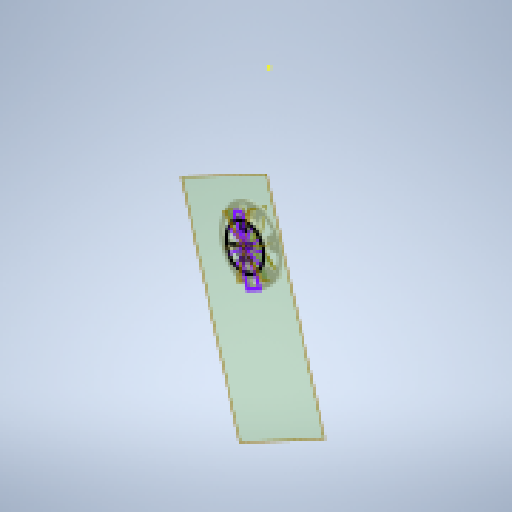
# Autodesk Inventor part: Part48
Saved by Autodesk Inventor 2023.1 (Build 271208000, 208)
## iProperties
Created: 2022-12-24
Part Number: Part48
Material: Generic
Document SubType Name: Modeling
Designer: USER
Density: 1 g/cm^3
Appearance: Default
Author: USER
## iProperties of the stored document Part48_3DPrint.ipt
Created: 2022-12-24
Part Number: Part48_3DPrint
Material: Generic
Document SubType Name: Modeling
Designer: USER
Density: 1 g/cm^3
Appearance: Default
Author: USER
Autodesk Inventor part; units mm, degrees
ref_plane "YZ Plane" through (0, 0, 0) normal (1, 0, 0) x (0, 1, 0)
ref_plane "XZ Plane" through (0, 0, 0) normal (0, 1, 0) x (-1, 0, 0)
ref_plane "XY Plane" through (0, 0, 0) normal (0, 0, 1) x (1, 0, 0)
ref_plane "Work Plane1" through (4.516, -244.3123, 193.8348) normal (0.0815899, -0.1423035, -0.9864547) x (-0.8818057, -0.4715874, -0.0049043)
sketch "Sketch1" plane through (4.516, -244.3123, 193.8348) normal (0.0815899, -0.1423035, -0.9864547) x (-0.8818057, -0.4715874, -0.0049043)
  circle A0 centre (-7.3856, 63.5963) radius 27.5
  circle A1 centre (-7.3856, 63.5963) radius 29.5
  line L0 (-7.3856, 63.5963) -> (21.2381, 70.733)
  line L1 (-7.3856, 63.5963) -> (22.1144, 63.5963) construction
  line L2 (-7.3856, 63.5963) -> (21.2381, 56.4596)
  line L3 (-7.3856, 63.5963) -> (-36.0093, 56.4596)
  line L4 (-7.3856, 63.5963) -> (11.5206, 86.2415)
  line L5 (-7.3856, 63.5963) -> (13.8349, 43.1038)
  line L6 (-7.3856, 63.5963) -> (-27.8852, 42.3827)
  line L7 (-7.3856, 63.5963) -> (-27.3405, 85.323)
  line L8 (-7.3856, 63.5963) -> (-36.0093, 70.733)
  line L9 (1.9118, 35.5997) -> (-7.3856, 63.5963)
  line L10 (-7.3856, 63.5963) -> (-14.5223, 34.9725)
  line L11 (-7.3856, 63.5963) -> (-3.5711, 92.8486)
  line L12 (-7.3856, 63.5963) -> (-13.8284, 92.3841)
  line L13 (1.2815, 37.4978) -> (-3.8297, 90.8654)
  line L14 (-14.0384, 36.9131) -> (-13.3916, 90.4324)
  line L15 (1.2815, 37.4978) -> (1.2815, 20.7047)
  line L16 (1.2815, 20.7047) -> (-15.5202, 20.7047)
  line L17 (-15.5202, 20.7047) -> (-14.0384, 36.9131)
  line L18 (-16.0526, 37.4978) -> (-17.5191, 18.7055)
  line L19 (-17.5191, 18.7055) -> (4.7638, 18.7055)
  line L20 (4.7638, 18.7055) -> (3.3138, 38.263)
  line L21 (-3.5711, 92.8486) -> (-4.046, 99.2535)
  line L22 (-4.046, 99.2535) -> (-6.8936, 100.1817)
  line L23 (-6.8936, 100.1817) -> (-9.9321, 100.1817)
  line L24 (-9.9321, 100.1817) -> (-13.8284, 98.8878)
  line L25 (-13.8284, 98.8878) -> (-13.8284, 92.3841)
  line L26 (-15.3417, 92.0031) -> (-15.3417, 99.2535)
  line L27 (-15.3417, 99.2535) -> (-9.9193, 101.5782)
  line L28 (-9.9193, 101.5782) -> (-7.0854, 101.5782)
  line L29 (-7.0854, 101.5782) -> (-3.122, 101.2612)
  line L30 (-3.122, 101.2612) -> (-0.9428, 92.3841)
  point P0 (-110.2818, 246.4946)
  point P1 (-14.0384, 36.9131)
  point P2 (-13.3916, 90.4324)
  point P3 (-3.8297, 90.8654)
  point P4 (1.2815, 37.4978)
  point P5 (-25.9876, 83.85)
  point P6 (-34.0687, 70.2491)
  point P7 (-34.0687, 56.9434)
  point P8 (-26.4954, 43.8209)
  point P9 (12.3963, 44.4932)
  point P10 (19.2975, 56.9434)
  point P11 (19.2975, 70.2491)
  point P12 (10.2388, 84.7062)
  point P13 (-14.2225, 34.8995)
  point P14 (-16.2126, 35.4478)
  point P15 (3.4693, 36.1659)
  point P16 (1.2815, 35.3982)
  dimension "d1" = 59
  dimension "d0" = 55
  dimension "d2" = 14
  constraints: 62 end point, 6 point on circle, 5 point on line, 4 parallel, 3 horizontal, 2 vertical, 1 centre point, 1 coincident, 1 equal length, 17 other
  measures "d0" diameter of A0
  measures "d2" angle of L1 L0
extrude "Extrusion1" add sketch "Sketch1" along normal blind 4 contours L11 A1 L4 A0 | A0 L7 A1 L12 | L4 A1 L0 A0 | A0 L8 A1 L7 | L0 A1 L2 A0 | A0 L20 A1 L9 | L10 A1 L18 A0 | A0 L3 A1 L8 | L2 A1 L5 A0 | A0 L6 A1 L3 | L5 A1 L20 A0 | A0 L18 A1 L6
extrude "Extrusion2" add sketch "Sketch1" along normal blind 8 contours L11 A1 L4 A0 | A0 L7 A1 L12 | L0 A1 L2 A0 | A0 L20 A1 L9 | L10 A1 L18 A0 | A0 L3 A1 L8 | L5 A1 L20 A0 | A0 L18 A1 L6
ref_plane "Work Plane2" through (-18.1856, -186.0532, 179.4979) normal (0.9966606, 0.0148992, 0.0802847) x (-0.0815899, 0.1423035, 0.9864547)
sketch "Sketch3" plane through (5.1687, -245.4507, 185.9432) normal (0.0815899, -0.1423035, -0.9864547) x (0.8818057, 0.4715874, 0.0049043)
  arc A0 (36.0093, -70.733) -> (36.0093, -56.4596) centre (7.3856, -63.5963) ccw projected
  line L0 (36.0093, -56.4596) -> (34.0687, -56.9434) projected
  arc A1 (34.0687, -70.2491) -> (34.0687, -56.9434) centre (7.3856, -63.5963) ccw projected
  line L1 (34.0687, -70.2491) -> (36.0093, -70.733) projected
  arc A2 (26.4954, -43.8209) -> (14.0384, -36.9131) centre (7.3856, -63.5963) ccw projected
  line L2 (26.4954, -43.8209) -> (27.8852, -42.3827) projected
  arc A3 (27.8852, -42.3827) -> (14.5223, -34.9725) centre (7.3856, -63.5963) ccw projected
  line L3 (14.5223, -34.9725) -> (14.0384, -36.9131) projected
  arc A4 (13.8284, -92.3841) -> (27.3405, -85.323) centre (7.3856, -63.5963) ccw projected
  line L4 (27.3405, -85.323) -> (25.9876, -83.85) projected
  arc A5 (13.3916, -90.4324) -> (25.9876, -83.85) centre (7.3856, -63.5963) ccw projected
  line L5 (13.3916, -90.4324) -> (13.8284, -92.3841) projected
  arc A6 (-10.2388, -84.7062) -> (3.8297, -90.8654) centre (7.3856, -63.5963) ccw projected
  line L6 (-10.2388, -84.7062) -> (-11.5206, -86.2415) projected
  arc A7 (-11.5206, -86.2415) -> (3.5711, -92.8486) centre (7.3856, -63.5963) ccw projected
  line L7 (3.5711, -92.8486) -> (3.8297, -90.8654) projected
  arc A8 (-21.2381, -56.4596) -> (-21.2381, -70.733) centre (7.3856, -63.5963) ccw projected
  line L8 (-21.2381, -70.733) -> (-19.2975, -70.2491) projected
  arc A9 (-19.2975, -56.9434) -> (-19.2975, -70.2491) centre (7.3856, -63.5963) ccw projected
  line L9 (-19.2975, -56.9434) -> (-21.2381, -56.4596) projected
  arc A10 (-1.9118, -35.5997) -> (-13.8349, -43.1038) centre (7.3856, -63.5963) ccw projected
  line L10 (-13.8349, -43.1038) -> (-12.3963, -44.4932) projected
  arc A11 (-1.2815, -37.4978) -> (-12.3963, -44.4932) centre (7.3856, -63.5963) ccw projected
  line L11 (-1.2815, -37.4978) -> (-1.9118, -35.5997) projected
  circle A12 centre (7.3856, -63.5963) radius 42.2209
  line L12 (-13.8349, -43.1038) -> (-22.6179, -33.8911)
  arc A13 (-1.9118, -35.5997) -> (3.5711, -92.8486) centre (7.3856, -63.5963) ccw projected
  line L13 (-1.9118, -35.5997) -> (-1.9118, -22.4118)
  arc A14 (27.8852, -42.3827) -> (14.5223, -34.9725) centre (7.3856, -63.5963) ccw projected
  line L14 (14.5223, -34.9725) -> (14.5223, -21.9829)
  line L15 (27.8852, -42.3827) -> (37.2658, -33.7671)
  line L16 (36.0093, -56.4596) -> (48.3523, -53.3821)
  line L17 (36.0093, -70.733) -> (48.3523, -73.8104)
  line L18 (27.3405, -85.323) -> (35.9454, -94.692)
  line L19 (13.8284, -92.3841) -> (14.5223, -105.2096)
  line L20 (3.5711, -92.8486) -> (3.5711, -105.6445)
  line L21 (-11.5206, -86.2415) -> (-20.7695, -95.0589)
  line L22 (-21.2381, -70.733) -> (-33.9344, -72.2715)
  line L23 (-21.2381, -56.4596) -> (-33.5811, -53.3821)
  circle A15 centre (7.3856, -63.5963) radius 46.8447
  circle A16 centre (-7.8498, -97.5441) radius 2.1
  circle A17 centre (-30.2116, -64.0433) radius 2.1
  circle A18 centre (-13.2655, -31.9742) radius 2.1
  circle A19 centre (25.3852, -30.0564) radius 2.1
  circle A20 centre (45.1864, -63.6105) radius 2.1
  circle A21 centre (25.0924, -96.3018) radius 2.1
  circle A22 centre (25.0924, -96.3018) radius 1.65
  circle A23 centre (45.1864, -63.6105) radius 1.65
  circle A24 centre (25.3852, -30.0564) radius 1.65
  circle A25 centre (-13.2655, -31.9742) radius 1.65
  circle A26 centre (-30.2116, -64.0433) radius 1.65
  circle A27 centre (-7.8498, -97.5441) radius 1.65
  point P0 (110.2818, -246.4946)
  dimension "d31" = 3.3
  dimension "d32" = 3.3
  dimension "d33" = 3.3
  dimension "d34" = 3.3
  dimension "d35" = 3.3
  dimension "d36" = 3.3
  constraints: 24 end point, 13 centre point, 8 coincident, 2 parallel, 2 perpendicular, 2 point on line, 1 point on circle, 1 vertical, 26 other
  measures "d31" diameter of A22
  measures "d32" diameter of A23
  measures "d33" diameter of A24
  measures "d34" diameter of A25
  measures "d35" diameter of A26
  measures "d36" diameter of A27
ref_plane "Work Plane3" through (-18.1856, -186.0532, 179.4979) normal (-0.4645017, 0.8702615, -0.1639608) x (0.0815899, -0.1423035, -0.9864547)
ref_plane "Work Plane4" through (-18.5119, -185.484, 183.4438) normal (-0.5459087, -0.8344608, 0.075225) x (-0.0815899, 0.1423035, 0.9864547)
ref_plane "Work Plane5" through (-18.5119, -185.484, 183.4438) normal (0.9937194, -0.064436, 0.0914861) x (0.0815899, -0.1423035, -0.9864547)
ref_plane "Work Plane6" through (-18.1856, -186.0532, 179.4979) normal (0.4645017, -0.8702615, 0.1639608) x (0.0815899, -0.1423035, -0.9864547)
ref_plane "Work Plane7" through (-18.1856, -186.0532, 179.4979) normal (-0.6214967, -0.7810177, 0.0612635) x (0.0815899, -0.1423035, -0.9864547)
extrude "Extrusion7" add sketch "Sketch3" along normal blind 2.0625 contours L1 A1 L0 A0 | A0 L16 A12 L17 | A12 L19 A4 L18 | L15 A3 L14 A12 | A4 L5 A5 L4 | L2 A2 L3 A3 | A12 L21 A7 L20 | L13 A10 L12 A12 | A7 L6 A6 L7 | L11 A11 L10 A10 | A12 L23 A8 L22 | A8 L9 A9 L8 | A16 | A17 | A18 | A19 | A20 | A21 | A22 | A23 | A24 | A25 | A26 | A27
extrude "Extrusion8" add sketch "Sketch3" along normal blind 2.0625 contours A15
extrude "Extrusion9" cut sketch "Sketch3" along normal blind 2.0625 contours A22 | A23 | A24 | A25 | A26 | A27
fillet "Fillet1" radius 3.5875 8 edges at (22.4291, -198.6372, 179.5722) (23.0941, -176.3387, 176.4105) (-30.4342, -226.7696, 179.2582) (-49.1553, -214.9775, 176.0087) (-58.2409, -198.7054, 172.9098) (-57.2168, -172.666, 169.2381) (-7.0349, -146.2393, 169.5764) (13.6051, -158.5608, 173.061)
fillet "Fillet2" radius 2 6 edges at (-17.9558, -157.4259, 171.3323) (8.1541, -172.7106, 175.6968) (6.7397, -202.3275, 179.8523) (-20.1184, -215.7602, 179.5686) (-43.8725, -200.5342, 175.4075) (-40.8443, -168.684, 171.0633)
fillet "Fillet3" radius 1 2 edges at (-43.8689, -196.1119, 182.8796) (5.5816, -172.227, 183.5241)
fillet "Fillet4" radius 1 12 edges at (-25.23, -160.0843, 173.6168) (-26.0723, -157.8688, 178.8347) (-25.7337, -159.0599, 178.7377) (-34.4585, -163.2364, 178.6185) (-35.176, -162.2266, 178.7104) (-33.8628, -164.2167, 173.4989) (-13.9602, -212.6109, 187.4366) (-13.7874, -213.7456, 187.9115) (-13.5805, -213.0709, 182.2241) (-0.0327, -205.8234, 187.6094) (0.745, -206.6633, 188.0918) (0.2002, -206.355, 182.3951)
body "Solid1"
